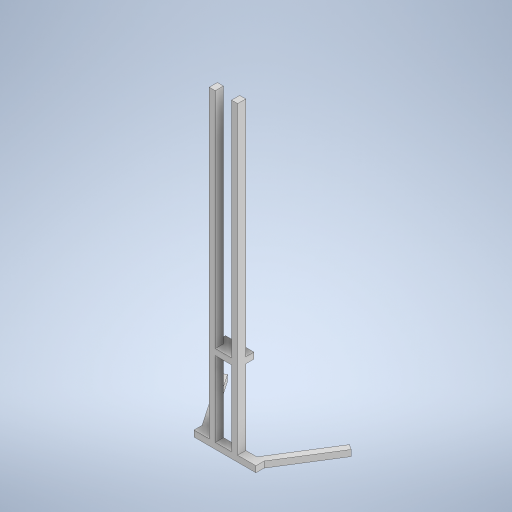
# Autodesk Inventor part: Стойка
Saved by Autodesk Inventor 2023 (Build 270158000, 158)
## iProperties
Created: 2022-05-29
Part Number: Стойка
Material: Типовые
Document SubType Name: Modeling
Designer: avkap
Density: 1 g/cm^3
Appearance: По умолчанию
Author: avkap
Autodesk Inventor part; units mm, degrees
ref_plane "YZ Plane" through (0, 0, 0) normal (1, 0, 0) x (0, 1, 0)
ref_plane "XZ Plane" through (0, 0, 0) normal (0, 1, 0) x (-1, 0, 0)
ref_plane "XY Plane" through (0, 0, 0) normal (0, 0, 1) x (1, 0, 0)
sketch "Эскиз1" plane through (0, 0, 0) normal (0, 0, 1) x (1, 0, 0)
  line L0 (0, 0) -> (110, 0)
  line L1 (0, 0) -> (15, 0)
  line L2 (15, 0) -> (-15, 0)
  line L3 (-15, 0) -> (-15, 1500)
  line L4 (-15, 1500) -> (15, 1500)
  line L5 (15, 1500) -> (15, 0)
  line L6 (110, 0) -> (95, 0)
  line L7 (95, 0) -> (125, 0)
  line L8 (125, 0) -> (125, 1500)
  line L9 (125, 1500) -> (95, 1500)
  line L10 (95, 1500) -> (95, 0)
  line L11 (0, 0) -> (-90, 0)
  line L12 (-90, 0) -> (-90, -30)
  line L13 (125, 0) -> (215, 0)
  line L14 (215, 0) -> (215, -30)
  line L15 (215, -30) -> (-90, -30)
  point P0 (-15, 0)
  dimension "d0" = 110
  dimension "d1" = 15
  dimension "d2" = 30
  dimension "d3" = 1500
  dimension "d4" = 15
  dimension "d5" = 30
  dimension "d6" = 1500
  dimension "d7" = 90
  dimension "d8" = 30
  dimension "d9" = 90
  constraints: 32 end point, 5 perpendicular, 4 parallel, 4 point on line, 3 horizontal
  measures "d0" distance of L0.start L0.end
  measures "d1" distance of L0.start L1.end
  measures "d2" distance of L3.end L4.end
  measures "d3" distance of L2.end L3.end
  measures "d4" distance of L0.end L6.end
  measures "d5" distance of L9.end L8.end
  measures "d6" distance of L8.end L7.end
  measures "d7" distance of L0.start L11.end
  measures "d8" distance of L11.end L12.end
  measures "d9" distance of L7.end L13.end
extrude "Выдавливание1" add sketch "Эскиз1" along normal blind 40
sketch "Эскиз2" plane through (-90, 0, 0) normal (0, 1, 0) x (1, 0, 0)
  line L0 (185, -40) -> (105, -40) projected
  line L1 (-191.3354, 280) -> (0, 0)
  line L2 (305, 0) -> (305, -40) projected
  line L3 (480.4002, 280) -> (305, 0)
  line L4 (445, 280) -> (269.5998, 0)
  line L5 (0, 0) -> (305, 0) projected
  line L6 (36.3354, 0) -> (-155, 280)
  line L7 (-191.3354, 280) -> (-155, 280)
  line L8 (445, 280) -> (480.4002, 280)
  line L9 (-155, 280) -> (445, 280)
  line L10 (0, 0) -> (0, -40) projected
  line L11 (0, 0) -> (36.3354, 0)
  line L12 (305, 0) -> (269.5998, 0)
  line L13 (305, 0) -> (215, 0) projected
  line L14 (185, 0) -> (105, 0) projected
  line L15 (145, 0) -> (145, 280)
  line L16 (270.8246, -0.1173) -> (29.7017, -0.1173)
  line L17 (-155, 280) -> (-179.7693, 263.0742)
  line L18 (445, 280) -> (470.4236, 264.0739)
  point P0 (90, 0)
  point P1 (269.5998, 0)
  dimension "d26" = 600
  dimension "d28" = 30
  dimension "d29" = 30
  constraints: 26 end point, 4 point on line, 3 perpendicular, 2 collinear, 2 horizontal, 2 midpoint, 1 parallel
  measures "d26" distance of L6.end L4.start
  measures "d28" distance between parallel lines of L3 L4
  measures "d29" distance between parallel lines of L6 L1
extrude "Выдавливание2" add sketch "Эскиз2" against normal blind 30 contours L17 L6 L5 L1 | L18 L3 L5 L4
sketch "Эскиз3" plane through (0, 0, 40) normal (0, 0, 1) x (1, 0, 0)
  line L0 (-15, 0) -> (-15, 400)
  line L1 (-15, 1500) -> (-15, 0) projected
  line L2 (-15, 400) -> (125, 400)
  line L3 (125, 0) -> (125, 1500) projected
  line L4 (125, 400) -> (125, 370)
  line L5 (125, 370) -> (-15, 370)
  point P0 (0, 0)
  point P1 (-15, 370)
  dimension "d22" = 400
  dimension "d23" = 30
  constraints: 8 end point, 3 point on line, 2 perpendicular, 1 horizontal
  measures "d22" distance of L0.start L0.end
  measures "d23" distance of L2.end L4.end
extrude "Выдавливание3" add sketch "Эскиз3" against normal blind 80
